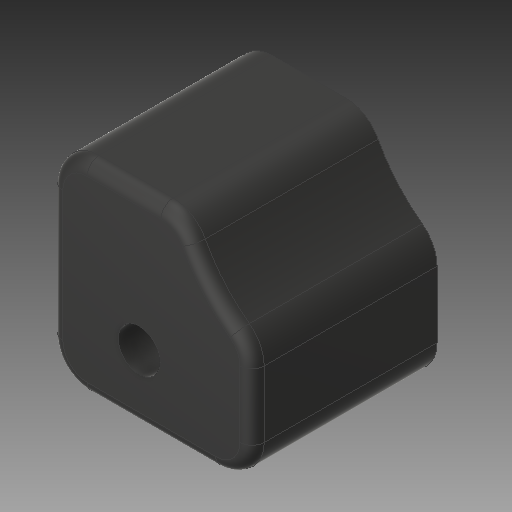
# Autodesk Inventor part: Spring Block
Saved by Autodesk Inventor 2018 (Build 220112000, 112)
## iProperties
Created: 2016-06-25
Part Number: Spring Block
Material: Acetal Resin, Black
Document SubType Name: Modeling
Designer: joshmamo
Density: 1.425 g/cm^3
Appearance: Smooth - Black
Mass: 5.04602 g
Surface Area: 15.9053 cm^2
Volume: 3.54106 cm^3
Author: joshmamo
Autodesk Inventor part; units mm, degrees
ref_plane "YZ Plane" through (0, 0, 0) normal (1, 0, 0) x (0, 1, 0)
ref_plane "XZ Plane" through (0, 0, 0) normal (0, 1, 0) x (-1, 0, 0)
sketch "Sketch1" plane through (0, 0, 0) normal (0, 0, 1) x (1, 0, 0)
  circle A0 centre (7.2868, -8.733) radius 1.7254
  line L0 (2.54, -14.1569) -> (14.054, -14.1569)
  line L1 (9.3709, 2.54) -> (2.54, 2.54)
  line L2 (16.594, -11.6169) -> (16.594, -5.4607)
  line L3 (0, 0) -> (0, -11.6169)
  arc A1 (11.744, 0.94) -> (15.3749, -3.2809) centre (22.7864, 6.7667) ccw
  line L4 (13.594, -14.1569) -> (3, -14.1569)
  line L5 (0, -11.1569) -> (0, -0.46)
  line L6 (3, 2.54) -> (9.3709, 2.54)
  line L7 (16.594, -5.6952) -> (16.594, -11.1569)
  arc A2 (11.744, 0.94) -> (15.3749, -3.2809) centre (22.7864, 6.7667) ccw
  arc A3 (13.594, -14.1569) -> (16.594, -11.1569) centre (13.594, -11.1569) ccw
  arc A4 (0, -11.1569) -> (3, -14.1569) centre (3, -11.1569) ccw
  arc A5 (3, 2.54) -> (0, -0.46) centre (3, -0.46) ccw
  line L8 (9.3709, 2.54) -> (9.0907, 2.54)
  arc A6 (16.594, -5.6952) -> (15.3749, -3.2809) centre (13.594, -5.6952) ccw
  arc A7 (11.744, 0.94) -> (9.0907, 2.54) centre (9.0907, -0.46) ccw
  point P0 (0, 0)
  point P1 (70.9762, -14.153)
  point P2 (11.0382, 2.54)
  dimension "d0" = 3
  dimension "d1" = 3
  constraints: 15 point on circle, 10 end point, 10 tangent, 9 point on line, 6 centre point, 4 equal radius, 3 collinear, 1 coincident, 1 perpendicular
  measures "d0" radius of A3
  measures "d1" radius of A6
ref_plane "Work Plane1" through (-2.8502, -20.8409, 15.24) normal (0, 0, 1) x (1, 0, 0)
extrude "Extrusion1" add sketch "Sketch1" along normal up to surface (15.24 mm away)
sketch "Sketch2" plane through (0, 0, 0) normal (0, 0, -1) x (-1, 0, 0)
  circle A0 centre (-7.2868, -8.733) radius 1.7254 projected
  line L0 (-9.0907, 2.54) -> (-3, 2.54) projected
  arc A1 (-9.0907, 2.54) -> (-11.744, 0.94) centre (-9.0907, -0.46) ccw projected
  arc A2 (-15.3749, -3.2809) -> (-11.744, 0.94) centre (-22.7864, 6.7667) ccw projected
  arc A3 (-15.3749, -3.2809) -> (-16.594, -5.6952) centre (-13.594, -5.6952) ccw projected
  line L1 (-16.594, -11.1569) -> (-16.594, -5.6952) projected
  arc A4 (-16.594, -11.1569) -> (-13.594, -14.1569) centre (-13.594, -11.1569) ccw projected
  line L2 (-3, -14.1569) -> (-13.594, -14.1569) projected
  arc A5 (-3, -14.1569) -> (0, -11.1569) centre (-3, -11.1569) ccw projected
  line L3 (0, -0.46) -> (0, -11.1569) projected
  arc A6 (0, -0.46) -> (-3, 2.54) centre (-3, -0.46) ccw projected
  line L4 (-13.594, -14.1569) -> (-3, -14.1569) projected
  line L5 (-4.6829, -13.2992) -> (-1.6998, -10.3864)
  line L6 (-1.6998, -10.3864) -> (-0.8807, -9.4246)
  line L7 (0, -9.7488) -> (0, -11.1569)
  line L8 (-4.3336, -14.1569) -> (-3, -14.1569)
  arc A7 (-4.6829, -13.2992) -> (-4.3336, -14.1569) centre (-4.3336, -13.6569) ccw
  arc A8 (0, -9.7488) -> (-0.8807, -9.4246) centre (-0.5, -9.7488) ccw
  point P0 (0, 0)
  point P1 (-5.5614, -14.1569)
  point P2 (0, -8.3905)
  dimension "d4" = 0.5
  constraints: 8 end point, 6 point on line, 4 point on circle, 4 tangent, 2 centre point, 1 collinear, 1 equal radius
  measures "d4" radius of A7
extrude "Extrusion2" add sketch "Sketch2" along normal blind 2 contours L3 A5 L2 A7 L5 L6 A8
sketch "Sketch3" plane through (3, -14.1569, 15.24) normal (0, -1, 0) x (1, 0, 0)
  line L0 (10.594, -15.24) -> (10.594, 0) projected
  line L1 (10.594, -7.62) -> (5.297, -7.62)
  line L2 (0, -17.24) -> (0, 0) projected
  circle A0 centre (5.297, -7.62) radius 4
  point P0 (-3, -15.24)
  dimension "d7" = 5.297
  dimension "d8" = 8
  constraints: 2 end point, 1 centre point, 1 coincident, 1 midpoint, 1 perpendicular
  measures "d7" distance of L1.start L1.end
  measures "d8" diameter of A0
extrude "Extrusion3" cut sketch "Sketch3" against normal blind 2
fillet "Fillet1" radius 1 10 edges at (0.8787, -13.2782, 15.24) (0, -5.8085, 15.24) (0.8787, 1.6613, 15.24) (6.0453, 2.54, 15.24) (10.6399, 2.1091, 15.24) (13.3211, -1.3754, 15.24) (16.272, -4.3429, 15.24) (16.594, -8.4261, 15.24) (15.7154, -13.2782, 15.24) (8.297, -14.1569, 15.24)
body "Solid1"
